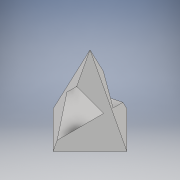
# Autodesk Inventor part: Пирамида
Saved by Autodesk Inventor 2017 (Build 210142000, 142)
## iProperties
Part Number: Пирамида
Material: Типовые
Document SubType Name: Modeling
Designer: 2000
Density: 1 g/cm^3
Appearance: По умолчанию
Author: 2000
Autodesk Inventor part; units mm, degrees
ref_plane "YZ Plane" through (0, 0, 0) normal (1, 0, 0) x (0, 1, 0)
ref_plane "XZ Plane" through (0, 0, 0) normal (0, 1, 0) x (-1, 0, 0)
sketch "Эскиз1" plane through (0, 0, 0) normal (0, 0, 1) x (1, 0, 0)
  point P0 (0, 0)
sketch "Эскиз2" plane through (0, 0, 0) normal (0, 0, 1) x (1, 0, 0)
  line L0 (0, 42.5) -> (42.5, 0)
  line L1 (42.5, 0) -> (0, -42.5)
  line L2 (0, -42.5) -> (-42.5, 0)
  line L3 (-42.5, 0) -> (0, 42.5)
  point P0 (0, 0)
  point P1 (0, 0)
  dimension "d0" = 85
  constraints: 8 end point, 1 coincident, 1 horizontal alignment, 9 other
  measures "d0" distance of L2.end L0.end
sketch "Эскиз3" plane through (0, 0, 0) normal (0, 0, 1) x (1, 0, 0)
  point P0 (0, 0)
ref_plane "РабПлоскость1" through (0, 0, 80) normal (0, 0, 1) x (1, 0, 0)
sketch "Эскиз4" plane through (0, 0, 80) normal (0, 0, 1) x (1, 0, 0)
  point P0 (0, 0)
loft "Лофт1" add profiles "Эскиз2" section 2 point at (0, 0, 80)
sketch "Эскиз5" plane through (0, 0, 0) normal (0, 1, 0) x (-1, 0, 0)
  line L0 (0, 8.7868) -> (-21.2132, 30)
  line L1 (-21.2132, 30) -> (0, 51.2132)
  line L2 (0, 51.2132) -> (21.2132, 30)
  line L3 (21.2132, 30) -> (0, 8.7868)
  line L4 (0, 0) -> (42.5, 0) projected
  point P0 (0, 30)
  dimension "d6" = 30
  dimension "d7" = 30
  constraints: 8 end point, 1 horizontal alignment, 1 vertical alignment, 9 other
  measures "d6" distance between parallel lines of L3 L1
  measures "d7" distance from line of L4 point (0, 30)
extrude "Выдавливание1" cut sketch "Эскиз5" along normal through all both and the other way through all
